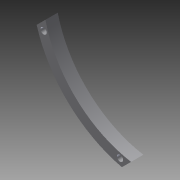
# Autodesk Inventor part: motor stay bottom
Saved by Autodesk Inventor 2012 (Build 160160000, 160)
## iProperties
Created: 2012-02-05
Part Number: motor stay bottom
Material: Default
Document SubType Name: Modeling
Designer: Antonella Wilby
Density: 1 g/cm^3
Author: Antonella Wilby
Autodesk Inventor part; units mm, degrees
ref_plane "YZ Plane" through (0, 0, 0) normal (1, 0, 0) x (0, 1, 0)
ref_plane "XZ Plane" through (0, 0, 0) normal (0, 1, 0) x (-1, 0, 0)
ref_plane "XY Plane" through (0, 0, 0) normal (0, 0, 1) x (1, 0, 0)
sketch "Sketch1" plane through (0, 0, 0) normal (0, 0, 1) x (1, 0, 0)
  line L0 (-86.8355, 0) -> (77.4434, 0) projected
  line L1 (0, -88.2763) -> (0, 77.6836) projected
  circle A0 centre (0, 0) radius 53.975 construction
  line L2 (-53.2759, -12.7) -> (-57.8106, -17.2347)
  line L3 (-9.2461, -53.9826) -> (-13.9527, -58.6892)
  arc A1 (-53.2759, -12.7) -> (-9.2461, -53.9826) centre (0, 0) ccw
  arc A2 (-57.8106, -17.2347) -> (-13.9527, -58.6892) centre (0, 0) ccw
  point P0 (-54.2025, -18.1167)
  point P1 (-14.9213, -55.1677)
  dimension "d16" = 107.95
  dimension "d17" = 60.325
  dimension "d18" = 5.5563
  dimension "d19" = 0.7937
  dimension "d20" = 3.175
  dimension "d21" = 3.175
  dimension "d22" = 57.15
  dimension "d23" = 57.15
  dimension "d24" = 45
  dimension "d25" = 12.7
  constraints: 4 end point, 4 point on circle, 3 centre point, 1 coincident, 1 parallel
  measures "d16" diameter of A0
  measures "d17" distance between parallel lines of L3 L2
  measures "d18" radial gap between concentric circles of A1 A2
  measures "d19" radial gap between concentric circles of A0 A1
  measures "d20" distance from line of L2 point (-54.202, -18.117)
  measures "d21" distance from line of point (-14.921, -55.168) L3
  measures "d22" distance of A0.centre point (-54.202, -18.117)
  measures "d23" distance of A0.centre point (-14.921, -55.168)
  measures "d24" angle of L0 L2
  measures "d25" distance from line of L0 L2.start
extrude "Extrusion1" add sketch "Sketch1" along normal blind 6.35
sketch "Sketch2" plane through (0, 0, 6.35) normal (0, 0, 1) x (1, 0, 0)
  circle A0 centre (0, 0) radius 53.975 construction
  arc A1 (-57.8106, -17.2347) -> (-13.9527, -58.6892) centre (0, 0) ccw projected
  line L0 (-57.8106, -17.2347) -> (-53.2759, -12.7) projected
  arc A2 (-53.2759, -12.7) -> (-9.2461, -53.9826) centre (0, 0) ccw projected
  line L1 (-9.2461, -53.9826) -> (-13.9527, -58.6892) projected
  line L2 (0, -88.9565) -> (0, 77.7969) projected
  line L3 (-87.5032, 0) -> (77.5547, 0) projected
  point P0 (-14.9213, -55.1677)
  point P1 (-54.2025, -18.1167)
  dimension "d27" = 107.95
  dimension "d33" = 57.15
  dimension "d34" = 57.15
  dimension "d37" = 3.175
  dimension "d38" = 3.175
  constraints: 1 centre point, 1 coincident
  measures "d27" diameter of A0
  measures "d33" distance of A0.centre point (-54.202, -18.117)
  measures "d34" distance of A0.centre point (-14.921, -55.168)
  measures "d37" distance from line of L0 point (-54.202, -18.117)
  measures "d38" distance from line of point (-14.921, -55.168) L1
hole "Hole1" at (-54.2025, -18.1167, 6.35) at (-14.9213, -55.1677, 6.35) direction (0, 0, -1) diameter 3.175 end through all
body "Solid1"
